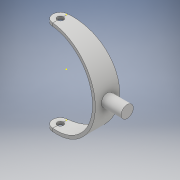
# Autodesk Inventor part: Sujetador Espejo
Saved by Autodesk Inventor 2018 (Build 220112000, 112)
## iProperties
Created: 2018-05-13
Part Number: Sujetador Espejo
Material: Generic
Document SubType Name: Modeling
Designer: Michel Gordillo
Density: 1 g/cm^3
Appearance: Default
Author: Michel Gordillo
Autodesk Inventor part; units mm, degrees
ref_plane "YZ Plane" through (0, 0, 0) normal (1, 0, 0) x (0, 1, 0)
ref_plane "XY Plane" through (0, 0, 0) normal (0, 0, 1) x (1, 0, 0)
sketch "Sketch1" plane through (0, 0, 0) normal (1, 0, 0) x (0, 1, 0)
  circle A0 centre (0, 0) radius 2
  dimension "d0" = 4
  constraints: 1 centre point, 1 coincident
  measures "d0" diameter of A0
extrude "Extrusion1" add sketch "Sketch1" along normal blind 7.5
ref_plane "Work Plane1" through (0, 2, 0) normal (0, 1, 0) x (-1, 0, 0)
sketch "Sketch2" plane through (0, 2, 0) normal (0, 1, 0) x (-1, 0, 0)
  arc A0 (14.5, 14.5) -> (14.5, -14.5) centre (14.5, 0) ccw
  arc A1 (14.5, 15.5) -> (14.5, -15.5) centre (14.5, 0) ccw
  line L0 (14.5, 15.5) -> (14.5, 14.5)
  line L1 (14.5, -14.5) -> (14.5, -15.5)
  point P0 (0, 0)
  dimension "d5" = 31
  constraints: 4 end point, 4 point on circle, 2 centre point, 2 point on line, 1 coincident, 1 vertical
  measures "d5" diameter of A1
extrude "Extrusion2" add sketch "Sketch2" against normal blind 4
sketch "Sketch3" plane through (0, 2, 0) normal (0, 1, 0) x (1, 0, 0)
  point P0 (-14.5, -14.5)
  point P1 (-14.5, 14.5)
  point P2 (-14.5, 0)
  point P3 (-14.5, -15.5)
ref_plane "Work Plane2" through (0, 4, 0) normal (0, 1, 0) x (-1, 0, 0)
sketch "Sketch4" plane through (0, 4, 0) normal (0, 1, 0) x (-1, 0, 0)
  arc A0 (14.5, 15.5) -> (-1, 0) centre (14.5, 0) ccw projected
  arc A1 (14.5, 15.5) -> (14.5, -15.5) centre (14.5, 0) ccw
  arc A2 (14.5, 14.5) -> (14.5, -14.5) centre (14.5, 0) ccw
  line L0 (14.5, 15.5) -> (14.5, 14.5)
  arc A3 (14.5, 14.5) -> (14.5, -14.5) centre (14.5, 0) ccw projected
  line L1 (14.5, -14.5) -> (14.5, -15.5)
  line L2 (14.5, 14.5) -> (17.5, 14.5)
  line L3 (17.5, 14.5) -> (17.5, 15.5)
  line L4 (17.5, 15.5) -> (14.5, 15.5)
  line L5 (14.5, -15.5) -> (17.5, -15.5)
  line L6 (17.5, -15.5) -> (17.5, -14.5)
  line L7 (17.5, -14.5) -> (14.5, -14.5)
  point P0 (0, 0)
  dimension "d10" = 3
  dimension "d11" = 1
  dimension "d12" = 3
  constraints: 16 end point, 5 point on circle, 3 perpendicular, 2 centre point, 2 coincident, 2 horizontal, 1 point on line
  measures "d10" distance of L0.end L2.end
  measures "d11" distance of L2.end L3.end
  measures "d12" distance of L1.end L5.end
extrude "Extrusion3" add sketch "Sketch4" against normal blind 8
sketch "Sketch5" plane through (-17.5, 4, 15.5) normal (0, 0, 1) x (1, 0, 0)
  line L0 (3, 0) -> (3, -8) projected
  circle A0 centre (3, -4) radius 2.5
  line L1 (3, -8) -> (18.5, -8) projected
  line L2 (3, -6.5) -> (18.5, -8)
  line L3 (18.5, -8) -> (-0.017, -8)
  line L4 (-0.017, -8) -> (-0.017, 0)
  line L5 (-0.017, 0) -> (18.5, 0)
  line L6 (18.5, 0) -> (18.5, -8) projected
  line L7 (18.5, 0) -> (3, -1.5)
  point P0 (17.5, -4)
  dimension "d15" = 5
  constraints: 10 end point, 3 point on line, 2 perpendicular, 2 point on circle, 1 centre point, 1 collinear, 1 midpoint
  measures "d15" diameter of A0
extrude "Extrusion4" cut sketch "Sketch5" against normal through all contours L5 L7 L0 | L0 A0 L3 L4 L5 | L2 L1 L0
sketch "Sketch6" plane through (-14.5, 0, -15.5) normal (0, 0, -1) x (-1, 0, 0)
  line L0 (0, 2.5) -> (0, -2.5) projected
  circle A0 centre (0, 0) radius 1
  point P0 (-14.5, 0)
  dimension "d18" = 2
  constraints: 1 centre point, 1 midpoint
  measures "d18" diameter of A0
extrude "Extrusion5" cut sketch "Sketch6" against normal through all
body "Solid1"
